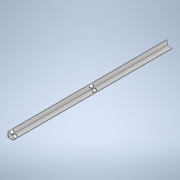
# Autodesk Inventor part: corner90
Saved by Autodesk Inventor 2020.2 (Build 242310000, 310)
## iProperties
Created: 2020-04-20
Part Number: corner90
Material: Generic
Document SubType Name: Modeling
Designer: Adam Nagy
Density: 1 g/cm^3
Appearance: Default
Author: Adam Nagy
Autodesk Inventor part; units mm, degrees
ref_plane "YZ Plane" through (0, 0, 0) normal (1, 0, 0) x (0, 1, 0)
ref_plane "XZ Plane" through (0, 0, 0) normal (0, 1, 0) x (-1, 0, 0)
ref_plane "XY Plane" through (0, 0, 0) normal (0, 0, 1) x (1, 0, 0)
sketch "Sketch1" plane through (0, 0, 0) normal (0, 0, 1) x (1, 0, 0)
  line L0 (0, 0) -> (30, 0)
  line L1 (30, 0) -> (30, 3)
  line L2 (30, 3) -> (3, 3)
  line L3 (3, 3) -> (3, 30)
  line L4 (3, 30) -> (0, 30)
  line L5 (0, 30) -> (0, 0)
  dimension "d0" = 3
  dimension "d1" = 3
  dimension "d2" = 30
  dimension "d3" = 30
  constraints: 12 end point, 5 perpendicular, 1 horizontal
  measures "d0" distance between parallel lines of L0 L2
  measures "d1" distance between parallel lines of L5 L3
  measures "d2" distance between parallel lines of L0 L4
  measures "d3" distance between parallel lines of L1 L5
extrude "Extrusion1" add sketch "Sketch1" along normal blind 900
sketch "Sketch2" plane through (3, 3, 900) normal (0, 1, 0) x (1, 0, 0)
  line L0 (0, 900) -> (0, 0) projected
  line L1 (27, 0) -> (0, 0) projected
  point P0 (-3, 900)
  point P1 (15, 15)
  point P2 (15, 465)
  point P3 (15, 915)
  point P4 (15, 1365)
  dimension "d6" = 15
  dimension "d7" = 15
  dimension "d8" = 27
  dimension "d9" = 15
  dimension "d10" = 450
  dimension "d11" = 450
  dimension "d12" = 15
  dimension "d13" = 450
  dimension "d14" = 15
  measures "d6" distance from line of point (15, 15) L0
  measures "d7" distance from line of point (15, 15) L1
  measures "d8" distance of L1.start L0.end
  measures "d9" distance from line of point (15, 465) L0
  measures "d10" distance of point (15, 15) point (15, 465)
  measures "d11" distance of point (15, 465) point (15, 915)
  measures "d12" distance from line of L0 point (15, 915)
  measures "d13" distance of point (15, 1365) point (15, 915)
  measures "d14" distance from line of L0 point (15, 1365)
hole "Hole1" at (18, 3, 885) at (18, 3, 435) at (18, 3, -15) at (18, 3, -465) direction (0, -1, 0) diameter 3.81 end through all
sketch "Sketch3" plane through (3, 30, 900) normal (1, 0, 0) x (0, 0, -1)
  line L0 (0, -27) -> (0, 0) projected
  line L1 (900, -27) -> (0, -27) projected
  point P0 (900, -30)
  point P1 (15, -12)
  point P2 (465, -12)
  point P3 (915, -12)
  point P4 (1365, -12)
  dimension "d22" = 15
  dimension "d23" = 15
  dimension "d24" = 15
  dimension "d25" = 450
  dimension "d26" = 450
  dimension "d27" = 15
  dimension "d28" = 450
  dimension "d29" = 15
  measures "d22" distance from line of point (15, -12) L0
  measures "d23" distance from line of point (15, -12) L1
  measures "d24" distance from line of point (465, -12) L1
  measures "d25" distance of point (465, -12) point (15, -12)
  measures "d26" distance of point (915, -12) point (465, -12)
  measures "d27" distance from line of L1 point (915, -12)
  measures "d28" distance of point (915, -12) point (1365, -12)
  measures "d29" distance from line of L1 point (1365, -12)
hole "Hole2" at (3, 18, 885) at (3, 18, 435) at (3, 18, -15) at (3, 18, -465) direction (-1, 0, 0) diameter 3.81 end through all
equation "\"d0\" = Thickness"
equation "\"d1\" = Thickness"
equation "\"d2\" = Width"
equation "\"d3\" = Width"
equation "\"d4\" = Height"
equation "\"d6\" = HoleDistance"
equation "\"d7\" = HoleDistance"
equation "\"d9\" = HoleDistance"
equation "\"d12\" = HoleDistance"
equation "\"d14\" = HoleDistance"
equation "\"d22\" = HoleDistance"
equation "\"d23\" = HoleDistance"
equation "\"d24\" = HoleDistance"
equation "\"d27\" = HoleDistance"
equation "\"d29\" = HoleDistance"
equation "\"Width\" = 30"
equation "\"Thickness\" = 3"
equation "\"Height\" = 900"
equation "\"HoleDistance\" = 15"
body "Solid1"
